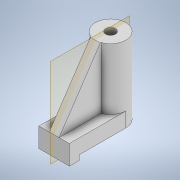
# Autodesk Inventor part: Pi3B_spacer_F
Saved by Autodesk Inventor 2022 (Build 260153000, 153)
## iProperties
Created: 2023-01-27
Part Number: Pi3B_spacer_F
Material: Generic
Document SubType Name: Modeling
Designer: scott
Density: 1 g/cm^3
Appearance: Default
Author: scott
Autodesk Inventor part; units mm, degrees
ref_plane "YZ Plane" through (0, 0, 0) normal (1, 0, 0) x (0, 1, 0)
ref_plane "XZ Plane" through (0, 0, 0) normal (0, 1, 0) x (-1, 0, 0)
ref_plane "XY Plane" through (0, 0, 0) normal (0, 0, 1) x (1, 0, 0)
sketch "Sketch1" plane through (0, 0, 0) normal (0, 1, 0) x (-1, 0, 0)
  line L0 (0, 0) -> (6.2, 0)
  line L1 (6.2, 0) -> (6.2, 9.5)
  line L2 (6.2, 9.5) -> (0, 9.5)
  line L3 (0, 9.5) -> (0, 0)
  circle A0 centre (3.1, 0) radius 3.1
  circle A1 centre (3.1, 0) radius 1
  dimension "d2" = 6.2
  dimension "d3" = 9.5
  dimension "d4" = 2
  constraints: 8 end point, 2 parallel, 1 centre point, 1 coincident, 1 horizontal, 1 midpoint, 1 perpendicular, 3 other
  measures "d2" distance of L2.end L1.end
  measures "d3" distance of L1.end L0.end
  measures "d4" diameter of A1
extrude "Extrusion1" add sketch "Sketch1" along normal blind 3 contours A1 L0 A0 | L0 A0 A1 | A0 L3 L2 L1
sketch "Sketch2" plane through (0, 3, 0) normal (0, 1, 0) x (1, 0, 0)
  circle A0 centre (-3.1, 0) radius 1 projected
  line L0 (-6.2, 0) -> (-6.2, -9.5) projected
  circle A1 centre (-3.1, 0) radius 3.1
  circle A2 centre (-3.1, 0) radius 1
  point P0 (0, 0)
  constraints: 2 coincident, 1 centre point, 1 concentric, 1 horizontal alignment, 2 other
extrude "Extrusion2" add sketch "Sketch2" along normal blind 12.5
sketch "Sketch3" plane through (0, 3, 0) normal (0, 1, 0) x (1, 0, 0)
  line L0 (-6.2, -9.5) -> (0, -9.5) projected
  line L1 (-6.2, -9.5) -> (0, -9.5)
  line L2 (0, -9.5) -> (0, -11.5)
  line L3 (0, -11.5) -> (-6.2, -11.5)
  line L4 (-6.2, -11.5) -> (-6.2, -9.5)
  point P0 (0, 0)
  dimension "d9" = 2
  constraints: 8 end point, 2 parallel, 1 horizontal, 1 perpendicular
  measures "d9" distance of L1.end L2.end
extrude "Extrusion3" add sketch "Sketch3" against normal blind 4
ref_plane "Work Plane1" through (-3.1, 0, 0) normal (1, 0, 0) x (0, 0, -1)
sketch "Sketch4" plane through (-3.1, 0, 0) normal (1, 0, 0) x (0, 0, -1)
  line L0 (-11.5, 3) -> (0, 3) projected
  line L1 (3.1, 15.5) -> (-3.1, 15.5) projected
  line L2 (-11.5, 3) -> (-3.1, 15.5)
  line L3 (-1, 15.5) -> (1, 15.5) projected
  line L4 (-3.1, 15.5) -> (-1, 15.5)
  line L5 (-1, 15.5) -> (-1, 3)
  line L6 (-11.5, 3) -> (-11.5, -1) projected
  line L7 (-1, 3) -> (-11.5, 3)
  point P0 (0, 0)
  constraints: 8 end point, 2 perpendicular, 1 collinear
extrude "Extrusion4" add sketch "Sketch4" along normal mid plane 2
body "Solid1"
